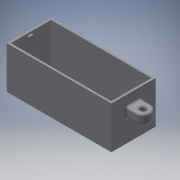
# Autodesk Inventor part: Casing_Part1
Saved by Autodesk Inventor 2019 (Build 230136000, 136)
## iProperties
Created: 2020-12-20
Part Number: Casing_Part1
Material: Generic
Document SubType Name: Modeling
Designer: nicolas
Density: 1 g/cm^3
Appearance: Default
Length: 100.000 mm
Width: 40.000 mm
Thickness: 2.000 mm
Depth: 40.000 mm
Author: nicolas
Autodesk Inventor part; units mm, degrees
ref_plane "YZ Plane" through (0, 0, 0) normal (1, 0, 0) x (0, 1, 0)
ref_plane "XZ Plane" through (0, 0, 0) normal (0, 1, 0) x (-1, 0, 0)
ref_plane "XY Plane" through (0, 0, 0) normal (0, 0, 1) x (1, 0, 0)
sketch "Sketch1" plane through (0, 0, 0) normal (0, 1, 0) x (-1, 0, 0)
  line L0 (0, 0) -> (-100, 0)
  line L1 (-100, 0) -> (-100, -40)
  line L2 (-100, -40) -> (0, -40)
  line L3 (0, -40) -> (0, 0)
  line L4 (2, -42) -> (-102, -42)
  line L5 (-102, -42) -> (-102, 2)
  line L6 (-102, 2) -> (2, 2)
  line L7 (2, 2) -> (2, -42)
  dimension "Length" = 100
  dimension "Width" = 40
  dimension "Thickness" = 2
  constraints: 16 end point, 4 parallel, 2 perpendicular, 1 horizontal, 3 other
  measures "Length" distance of L1.end L2.end
  measures "Width" distance of L0.end L1.end
  measures "Thickness" distance between parallel lines of L2 L4
extrude "Extrusion1" add sketch "Sketch1" along normal blind 40
sketch "Sketch2" plane through (0, 0, 0) normal (0, -1, 0) x (1, 0, 0)
  line L0 (102, -42) -> (102, 2) projected
  line L1 (102, 2) -> (-2, 2) projected
  line L2 (-2, -42) -> (102, -42) projected
  line L3 (-2, 2) -> (-2, -42) projected
  point P0 (0, 0)
extrude "Extrusion2" add sketch "Sketch2" along normal blind 2
sketch "Sketch3" plane through (-2, 40, -42) normal (-1, 0, 0) x (0, 0, 1)
  line L0 (0, 0) -> (44, 0) projected
  line L1 (19.5, -4) -> (24.5, -4)
  line L2 (24.5, -4) -> (24.5, -2)
  line L3 (24.5, -2) -> (19.5, -2)
  line L4 (19.5, -2) -> (19.5, -4)
  line L5 (19.5, -4) -> (24.5, -2) construction
  line L6 (24.5, -4) -> (19.5, -2) construction
  line L7 (22, -3) -> (22, 0) construction
  point P0 (42, -40)
  dimension "d7" = 5
  dimension "d8" = 2
  dimension "d9" = 2
  constraints: 14 end point, 3 midpoint, 2 parallel, 1 horizontal, 1 perpendicular, 1 vertical
  measures "d7" distance of L3.end L2.end
  measures "d8" distance of L2.end L1.end
  measures "d9" distance between parallel lines of L0 L3
extrude "Extrusion3" cut sketch "Sketch3" against normal up to next
sketch "Sketch4" plane through (102, 40, 2) normal (1, 0, 0) x (0, 0, -1)
  line L0 (14.5, -12) -> (29.5, -12)
  line L1 (29.5, -12) -> (29.5, -10)
  line L2 (29.5, -10) -> (14.5, -10)
  line L3 (14.5, -10) -> (14.5, -12)
  line L4 (14.5, -12) -> (29.5, -10) construction
  line L5 (29.5, -12) -> (14.5, -10) construction
  line L6 (0, 0) -> (44, 0) projected
  line L7 (22, -11) -> (22, 0) construction
  line L8 (44, 0) -> (0, 0) projected
  point P0 (2, -40)
  dimension "d12" = 10
  dimension "d13" = 15
  dimension "d14" = 2
  constraints: 14 end point, 3 midpoint, 2 parallel, 1 horizontal, 1 perpendicular, 1 vertical
  measures "d12" distance between parallel lines of L6 L2
  measures "d13" distance of L1.end L2.end
  measures "d14" distance of L0.end L1.end
extrude "Extrusion4" add sketch "Sketch4" along normal blind 10
sketch "Sketch5" plane through (102, 30, -12.5) normal (0, 1, 0) x (1, 0, 0)
  line L0 (0, 0) -> (0, 15) projected
  line L1 (0, 0) -> (10, 0) projected
  line L2 (10, 15) -> (10, 0) projected
  line L3 (0, 15) -> (10, 15) projected
  line L4 (10, 0) -> (10, 15) projected
  arc A0 (10, 0) -> (10, 15) centre (10, 7.5) ccw
  point P0 (-102, -12.5)
  constraints: 2 end point, 2 point on circle, 1 centre point, 1 midpoint
extrude "Extrusion5" add sketch "Sketch5" against normal blind 10
sketch "Sketch6" plane through (102, 30, -12.5) normal (0, 1, 0) x (1, 0, 0)
  arc A0 (10, 0) -> (10, 15) centre (10, 7.5) ccw projected
  point P0 (-102, -12.5)
hole "Hole1" at (112, 30, -20) direction (0, -1, 0) diameter 5.5 end through all clearance for "Countersunk Flat Head Screw ISO 2009/7046" size "M5" standard "ISO"
fillet "Fillet1" radius 2 11 edges at (119.5, 30, -20) (107, 30, -12.5) (107, 30, -27.5) (112, 30, -22.75) (119.5, 20, -20) (107, 20, -12.5) (107, 20, -27.5) (102, 25, -27.5) (102, 20, -20) (102, 25, -12.5) (102, 30, -20)
sketch "Sketch7" plane through (102, 20, -12.5) normal (0, -1, 0) x (1, 0, 0)
  circle A0 centre (10, -7.5) radius 2.75 projected
  circle A1 centre (10, -7.5) radius 4 construction
  line L0 (14, -9.8094) -> (10, -12.1188)
  line L1 (10, -12.1188) -> (6, -9.8094)
  line L2 (6, -9.8094) -> (6, -5.1906)
  line L3 (6, -5.1906) -> (10, -2.8812)
  line L4 (10, -2.8812) -> (14, -5.1906)
  line L5 (14, -5.1906) -> (14, -9.8094)
  point P0 (-102, 12.5)
  point P1 (14, -7.5)
  dimension "d27" = 8
  constraints: 12 end point, 2 coincident, 1 horizontal alignment, 1 midpoint, 1 vertical, 15 other
extrude "Extrusion6" cut sketch "Sketch7" against normal blind 3.5
equation "\"d5\" = Thickness"
equation "\"d10\" = Thickness"
equation "\"d14\" = Thickness"
body "Solid1"
